obudowa v5 (Autodesk Fusion 360 design; units mm, degrees)
Autodesk Fusion 360 part; units mm, degrees
note: some values were not read from the file. Set by a fixed rule: which sketch regions a step uses.
sketch "Sketch1" plane through (0, 0, 0) normal (0, 0, 1) x (1, 0, 0)
  circle A0 centre (0, 0) radius 28.5
  circle A1 centre (0, 0) radius 25 construction
  circle A2 centre (0.0994, 24.9998) radius 3 construction
  circle A3 centre (0, 0) radius 30
  dimension "d1" = 57
  dimension "d11" = 50
  dimension "d12" = 6
  dimension "d16" = 60
  constraint coincident A0.centre A1.centre
  constraint coincident A1 A2.centre
  measures "d1" diameter of A0
  measures "d11" diameter of A1
  measures "d12" diameter of A2
  measures "d16" diameter of A3
extrude "Extrude1" add sketch "Sketch1" along normal blind 26
sketch "Sketch2" plane through (0, 0, 26) normal (0, 0, 1) x (-1, 0, 0)
  circle A0 centre (0, 0) radius 28.5
  line L0 (0, 0) -> (-40, 0) construction
  line L1 (0, 0) -> (0, -30.5) construction
  circle A1 centre (-35, 0) radius 2.75
  line L2 (-29.5804, -5) -> (-40, -5)
  line L3 (-40, -5) -> (-40, 5)
  line L4 (-40, 5) -> (-29.5804, 5)
  line L5 (29.5804, -5) -> (40, -5)
  circle A2 centre (35, 0) radius 2.75
  line L6 (40, -5) -> (40, 5)
  line L7 (40, 5) -> (29.5804, 5)
  circle A3 centre (0, 0) radius 30
  dimension "d7" = 5.5
  dimension "d8" = 10
  dimension "d9" = 5
  dimension "d13" = 35
  constraint coincident A0.centre L0.start
  constraint horizontal L0
  constraint perpendicular L0 L1
  constraint coincident L0 A1.centre
  constraint horizontal L2
  constraint perpendicular L2 L3
  constraint perpendicular L3 L4
  constraint symmetric L0 L2 L4
  constraint midpoint L0.end L3
  constraint symmetric L1 A1 A2
  constraint symmetric L1 L2.start L5.start
  constraint symmetric L1 L2.end L5.end
  constraint symmetric L1 L3.end L6.end
  constraint symmetric L1 L4.end L7.end
  constraint coincident L2.start A3
  constraint coincident L4.end A3
  measures "d7" diameter of A1
  measures "d8" distance of L2.end L3.end
  measures "d9" distance of A1.centre L3
  measures "d13" distance of A0.centre A1.centre
extrude "Extrude2" add sketch "Sketch2" against normal blind 26 contours L2 L3 L4 A3 | L5 L6 L7 A3
